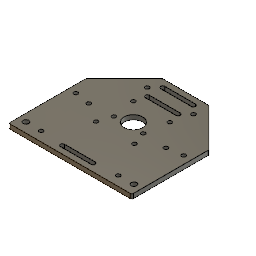
Motor_Mounting_Plate (Autodesk Fusion 360 design; units mm, degrees)
Autodesk Fusion 360 part; units mm, degrees
sketch "Sketch16" plane through (0, 0, 0) normal (0, 1, 0) x (1, 0, 0)
sketch "Sketch1" plane through (0, 0, 0) normal (0, 1, 0) x (1, 0, 0)
  line L0 (0, 0) -> (160, 0)
  line L1 (160, 0) -> (160, -150)
  line L2 (160, -150) -> (0, -150)
  line L3 (0, -150) -> (0, 0)
  line L4 (0, 0) -> (50, 0)
  line L5 (160, 0) -> (110, 0)
  line L6 (0, 0) -> (0, -50)
  line L7 (160, 0) -> (160, -50)
  line L8 (0, -50) -> (50, 0)
  line L9 (110, 0) -> (160, -50)
  dimension "d1" = 160
  dimension "d2" = 150
  dimension "d3" = 50
  dimension "d4" = 50
  dimension "d5" = 50
  measures "d1" distance of L0.start L0.end
  measures "d2" distance of L0.start L2.end
  measures "d3" distance of L0.end L5.end
  measures "d4" distance of L0.start L6.end
  measures "d5" distance of L0.end L7.end
extrude "Extrude1" add sketch "Sketch1" along normal blind 10 contours L0 L1 L2 L3 L8 L9
sketch "Sketch2" plane through (0, 10, 0) normal (0, 1, 0) x (-1, 0, 0)
  line L0 (-110, 0) -> (-50, 0)
  line L1 (-50, 0) -> (0, 50)
  line L2 (0, 50) -> (0, 150)
  line L3 (0, 150) -> (-160, 150)
  line L4 (-160, 150) -> (-160, 50)
  line L5 (-160, 50) -> (-110, 0)
  line L6 (0, 50) -> (-160, 50)
  line L7 (-80, 0) -> (-80, 150)
  circle A0 centre (-10, 72.7) radius 2.625
  circle A1 centre (-150.0228, 72.7) radius 2.625
  dimension "d10" = 5.25
  dimension "d13" = 5.25
  measures "d10" diameter of A0
  measures "d13" diameter of A1
extrude "Extrude2" cut sketch "Sketch2" against normal blind 200 contours A0 | A1
sketch "Sketch3" plane through (0, 10, 0) normal (0, 1, 0) x (-1, 0, 0)
  circle A0 centre (-10, 72.7) radius 2.625
  circle A1 centre (-150.0228, 72.7) radius 2.625
  line L0 (-110, 0) -> (-50, 0)
  line L1 (-50, 0) -> (0, 50)
  line L2 (0, 50) -> (0, 150)
  line L3 (0, 150) -> (-160, 150)
  line L4 (-160, 150) -> (-160, 50)
  line L5 (-160, 50) -> (-110, 0)
  line L6 (-80, 150) -> (-80, 68)
  circle A2 centre (-80, 68) radius 12
  dimension "d16" = 82
  dimension "d17" = 24
  measures "d16" distance of L6.start L6.end
  measures "d17" diameter of A2
extrude "Extrude3" cut sketch "Sketch3" against normal blind 45 contours A2
sketch "Sketch4" plane through (0, 10, 0) normal (0, 1, 0) x (-1, 0, 0)
  circle A0 centre (-80, 68) radius 12
  circle A1 centre (-10, 72.7) radius 2.625
  circle A2 centre (-150.0228, 72.7) radius 2.625
  line L0 (-110, 0) -> (-50, 0)
  line L1 (-50, 0) -> (0, 50)
  line L2 (0, 50) -> (0, 150)
  line L3 (0, 150) -> (-160, 150)
  line L4 (-160, 150) -> (-160, 50)
  line L5 (-160, 50) -> (-110, 0)
  line L6 (0, 150) -> (-30, 150)
  line L7 (-30, 150) -> (-30, 20)
  line L8 (-30, 150) -> (-30, 75.8)
  circle A3 centre (-30, 75.8) radius 2.625
  dimension "d20" = 30
  dimension "d21" = 130
  dimension "d22" = 74.2
  dimension "d23" = 5.25
  measures "d20" distance of L2.end L6.end
  measures "d21" distance of L6.end L7.end
  measures "d22" distance of L6.end L8.end
  measures "d23" diameter of A3
extrude "Extrude4" cut sketch "Sketch4" against normal blind 20 contours L7 L8 A3 | L7 L8 A3
sketch "Sketch5" plane through (0, 10, 0) normal (0, 1, 0) x (-1, 0, 0)
  circle A0 centre (-30, 75.8) radius 2.625
  circle A1 centre (-80, 68) radius 12
  circle A2 centre (-10, 72.7) radius 2.625
  circle A3 centre (-150.0228, 72.7) radius 2.625
  line L0 (-110, 0) -> (-50, 0)
  line L1 (-50, 0) -> (0, 50)
  line L2 (0, 50) -> (0, 150)
  line L3 (0, 150) -> (-160, 150)
  line L4 (-160, 150) -> (-160, 50)
  line L5 (-160, 50) -> (-110, 0)
  line L6 (0, 150) -> (-10, 150)
  line L7 (-10, 150) -> (-10, 137.3)
  line L8 (-160, 150) -> (-150, 150)
  line L9 (-150, 150) -> (-150, 137.3)
  circle A4 centre (-150, 137.3) radius 3.5685
  circle A5 centre (-10, 137.3) radius 3.5685
  dimension "d26" = 12.7
  dimension "d27" = 10
  dimension "d28" = 12.7
  dimension "d29" = 7.137
  dimension "d30" = 7.137
  measures "d26" distance of L6.end L7.end
  measures "d27" distance of L3.end L8.end
  measures "d28" distance of L8.end L9.end
  measures "d29" diameter of A4
  measures "d30" diameter of A5
extrude "Extrude5" cut sketch "Sketch5" against normal blind 12 contours A4 | A5
sketch "Sketch6" plane through (0, 10, 0) normal (0, 1, 0) x (-1, 0, 0)
  circle A0 centre (-10, 137.3) radius 3.5685
  circle A1 centre (-150, 137.3) radius 3.5685
  circle A2 centre (-30, 75.8) radius 2.625
  circle A3 centre (-80, 68) radius 12
  circle A4 centre (-10, 72.7) radius 2.625
  circle A5 centre (-150.0228, 72.7) radius 2.625
  line L0 (-110, 0) -> (-50, 0)
  line L1 (-50, 0) -> (0, 50)
  line L2 (0, 50) -> (0, 150)
  line L3 (0, 150) -> (-160, 150)
  line L4 (-160, 150) -> (-160, 50)
  line L5 (-160, 50) -> (-110, 0)
  line L6 (0, 150) -> (-30, 150)
  line L7 (-160, 150) -> (-130, 150)
  line L8 (-130, 150) -> (-130, 137.53)
  line L9 (-30, 150) -> (-30, 137.53)
  circle A6 centre (-30, 137.53) radius 2.625
  circle A7 centre (-130, 137.53) radius 2.625
  dimension "d33" = 30
  dimension "d34" = 30
  dimension "d35" = 12.47
  dimension "d36" = 12.47
  dimension "d37" = 5.25
  dimension "d38" = 5.25
  measures "d33" distance of L2.end L6.end
  measures "d34" distance of L3.end L7.end
  measures "d35" distance of L7.end L8.end
  measures "d36" distance of L6.end L9.end
  measures "d37" diameter of A6
  measures "d38" diameter of A7
extrude "Extrude6" cut sketch "Sketch6" against normal blind 20 contours A6 | A7
sketch "Sketch7" plane through (0, 10, 0) normal (0, 1, 0) x (-1, 0, 0)
  circle A0 centre (-30, 137.53) radius 2.625
  circle A1 centre (-130, 137.53) radius 2.625
  circle A2 centre (-10, 137.3) radius 3.5685
  circle A3 centre (-150, 137.3) radius 3.5685
  circle A4 centre (-30, 75.8) radius 2.625
  circle A5 centre (-80, 68) radius 12
  circle A6 centre (-10, 72.7) radius 2.625
  circle A7 centre (-150.0228, 72.7) radius 2.625
  line L0 (-110, 0) -> (-50, 0)
  line L1 (-50, 0) -> (0, 50)
  line L2 (0, 50) -> (0, 150)
  line L3 (0, 150) -> (-160, 150)
  line L4 (-160, 150) -> (-160, 50)
  line L5 (-160, 50) -> (-110, 0)
  line L6 (-130, 137.53) -> (-130, 60)
  line L7 (-30, 75.8) -> (-130, 75.8)
  circle A8 centre (-130, 75.8) radius 2.625
  dimension "d41" = 5.25
  measures "d41" diameter of A8
extrude "Extrude7" cut sketch "Sketch7" against normal blind 20 contours L6 L7 A8 | L6 A8 | L6 L7 A8
sketch "Sketch8" plane through (0, 10, 0) normal (0, 1, 0) x (-1, 0, 0)
  circle A0 centre (-130, 75.8) radius 2.625
  circle A1 centre (-30, 137.53) radius 2.625
  circle A2 centre (-130, 137.53) radius 2.625
  circle A3 centre (-10, 137.3) radius 3.5685
  circle A4 centre (-150, 137.3) radius 3.5685
  circle A5 centre (-30, 75.8) radius 2.625
  circle A6 centre (-80, 68) radius 12
  circle A7 centre (-10, 72.7) radius 2.625
  circle A8 centre (-150.0228, 72.7) radius 2.625
  line L0 (-110, 0) -> (-50, 0)
  line L1 (-50, 0) -> (0, 50)
  line L2 (0, 50) -> (0, 150)
  line L3 (0, 150) -> (-160, 150)
  line L4 (-160, 150) -> (-160, 50)
  line L5 (-160, 50) -> (-110, 0)
  line L6 (-80, 68) -> (-80, 150)
  line L7 (0, 150) -> (-99, 150)
  line L8 (0, 150) -> (-61, 150)
  line L9 (-61, 150) -> (-61, 74.1)
  line L10 (-99, 150) -> (-99, 74.1)
  circle A9 centre (-61, 74.1) radius 2.625
  circle A10 centre (-99, 74.1) radius 2.625
  dimension "d44" = 99
  dimension "d45" = 61
  dimension "d46" = 75.9
  dimension "d47" = 75.9
  dimension "d48" = 5.25
  dimension "d49" = 5.25
  measures "d44" distance of L2.end L7.end
  measures "d45" distance of L2.end L8.end
  measures "d46" distance of L8.end L9.end
  measures "d47" distance of L7.end L10.end
  measures "d48" diameter of A9
  measures "d49" diameter of A10
extrude "Extrude8" cut sketch "Sketch8" against normal blind 35 contours A9 | A10
sketch "Sketch9" plane through (0, 10, 0) normal (0, 1, 0) x (-1, 0, 0)
  circle A0 centre (-61, 74.1) radius 2.625
  circle A1 centre (-99, 74.1) radius 2.625
  circle A2 centre (-130, 75.8) radius 2.625
  circle A3 centre (-30, 137.53) radius 2.625
  circle A4 centre (-130, 137.53) radius 2.625
  circle A5 centre (-10, 137.3) radius 3.5685
  circle A6 centre (-150, 137.3) radius 3.5685
  circle A7 centre (-30, 75.8) radius 2.625
  circle A8 centre (-80, 68) radius 12
  circle A9 centre (-10, 72.7) radius 2.625
  circle A10 centre (-150.0228, 72.7) radius 2.625
  line L0 (-110, 0) -> (-50, 0)
  line L1 (-50, 0) -> (0, 50)
  line L2 (0, 50) -> (0, 150)
  line L3 (0, 150) -> (-160, 150)
  line L4 (-160, 150) -> (-160, 50)
  line L5 (-160, 50) -> (-110, 0)
  line L6 (0, 55) -> (-56.43, 55)
  line L7 (0, 55) -> (-103.57, 55)
  line L8 (-56.43, 55) -> (-56.43, 155)
  line L9 (-103.57, 55) -> (-103.57, 164.8084)
  line L10 (-103.57, 150) -> (-103.57, 44.43)
  line L11 (-56.43, 150) -> (-56.43, 44.43)
  circle A11 centre (-56.43, 44.43) radius 2.625
  circle A12 centre (-103.57, 44.43) radius 2.625
  dimension "d52" = 56.43
  dimension "d53" = 103.57
  dimension "d54" = 100
  dimension "d55" = 105.57
  dimension "d56" = 105.57
  dimension "d57" = 5.25
  dimension "d58" = 5.25
  measures "d52" distance of L6.start L6.end
  measures "d53" distance of L6.start L7.end
  measures "d54" distance of L6.end L8.end
  measures "d55" distance of L10.start L10.end
  measures "d56" distance of L11.start L11.end
  measures "d57" diameter of A11
  measures "d58" diameter of A12
extrude "Extrude9" cut sketch "Sketch9" against normal blind 12 contours A11 | A12
sketch "Sketch10" plane through (0, 10, 0) normal (0, 1, 0) x (-1, 0, 0)
  circle A0 centre (-103.57, 44.43) radius 2.625
  circle A1 centre (-56.43, 44.43) radius 2.625
  circle A2 centre (-61, 74.1) radius 2.625
  circle A3 centre (-99, 74.1) radius 2.625
  circle A4 centre (-130, 75.8) radius 2.625
  circle A5 centre (-30, 137.53) radius 2.625
  circle A6 centre (-130, 137.53) radius 2.625
  circle A7 centre (-10, 137.3) radius 3.5685
  circle A8 centre (-150, 137.3) radius 3.5685
  circle A9 centre (-30, 75.8) radius 2.625
  circle A10 centre (-80, 68) radius 12
  circle A11 centre (-10, 72.7) radius 2.625
  circle A12 centre (-150.0228, 72.7) radius 2.625
  line L0 (-110, 0) -> (-50, 0)
  line L1 (-50, 0) -> (0, 50)
  line L2 (0, 50) -> (0, 150)
  line L3 (0, 150) -> (-160, 150)
  line L4 (-160, 150) -> (-160, 50)
  line L5 (-160, 50) -> (-110, 0)
  line L6 (0, 150) -> (-55, 150)
  line L7 (0, 150) -> (-105, 150)
  line L8 (-55, 150) -> (-55, 91.57)
  line L9 (-105, 150) -> (-105, 91.57)
  circle A13 centre (-55, 91.57) radius 2.625
  circle A14 centre (-105, 91.57) radius 2.625
  dimension "d61" = 55
  dimension "d62" = 105
  dimension "d63" = 58.43
  dimension "d64" = 58.43
  dimension "d65" = 5.25
  dimension "d66" = 5.25
  measures "d61" distance of L2.end L6.end
  measures "d62" distance of L2.end L7.end
  measures "d63" distance of L6.end L8.end
  measures "d64" distance of L7.end L9.end
  measures "d65" diameter of A13
  measures "d66" diameter of A14
extrude "Extrude10" cut sketch "Sketch10" against normal blind 12 contours A13 | A14
sketch "Sketch11" plane through (0, 0, 0) normal (0, 1, 0) x (1, 0, 0)
sketch "Sketch12" plane through (0, 10, 0) normal (0, 1, 0) x (-1, 0, 0)
  circle A0 centre (-105, 91.57) radius 2.625
  circle A1 centre (-55, 91.57) radius 2.625
  circle A2 centre (-103.57, 44.43) radius 2.625
  circle A3 centre (-56.43, 44.43) radius 2.625
  circle A4 centre (-61, 74.1) radius 2.625
  circle A5 centre (-99, 74.1) radius 2.625
  circle A6 centre (-130, 75.8) radius 2.625
  circle A7 centre (-30, 137.53) radius 2.625
  circle A8 centre (-130, 137.53) radius 2.625
  circle A9 centre (-10, 137.3) radius 3.5685
  circle A10 centre (-150, 137.3) radius 3.5685
  circle A11 centre (-30, 75.8) radius 2.625
  circle A12 centre (-80, 68) radius 12
  circle A13 centre (-10, 72.7) radius 2.625
  circle A14 centre (-150.0228, 72.7) radius 2.625
  line L0 (-110, 0) -> (-50, 0)
  line L1 (-50, 0) -> (0, 50)
  line L2 (0, 50) -> (0, 150)
  line L3 (0, 150) -> (-160, 150)
  line L4 (-160, 150) -> (-160, 50)
  line L5 (-160, 50) -> (-110, 0)
  line L6 (0, 150) -> (-50, 150)
  line L7 (-50, 150) -> (-50, 20)
  line L8 (0, 150) -> (-110, 150)
  line L9 (-110, 150) -> (-110, 20)
  circle A15 centre (-50, 20) radius 2.625
  circle A16 centre (-110, 20) radius 2.625
  dimension "d69" = 50
  dimension "d70" = 130
  dimension "d71" = 110
  dimension "d72" = 130
  dimension "d73" = 5.25
  dimension "d74" = 5.25
  measures "d69" distance of L2.end L6.end
  measures "d70" distance of L6.end L7.end
  measures "d71" distance of L2.end L8.end
  measures "d72" distance of L8.end L9.end
  measures "d73" diameter of A15
  measures "d74" diameter of A16
extrude "Extrude11" cut sketch "Sketch12" against normal blind 20 contours A15 | A16
sketch "Sketch13" plane through (0, 10, 0) normal (0, 1, 0) x (-1, 0, 0)
  circle A0 centre (-110, 20) radius 2.625
  circle A1 centre (-50, 20) radius 2.625
  circle A2 centre (-105, 91.57) radius 2.625
  circle A3 centre (-55, 91.57) radius 2.625
  circle A4 centre (-103.57, 44.43) radius 2.625
  circle A5 centre (-56.43, 44.43) radius 2.625
  circle A6 centre (-61, 74.1) radius 2.625
  circle A7 centre (-99, 74.1) radius 2.625
  circle A8 centre (-130, 75.8) radius 2.625
  circle A9 centre (-30, 137.53) radius 2.625
  circle A10 centre (-130, 137.53) radius 2.625
  circle A11 centre (-10, 137.3) radius 3.5685
  circle A12 centre (-150, 137.3) radius 3.5685
  circle A13 centre (-30, 75.8) radius 2.625
  circle A14 centre (-80, 68) radius 12
  circle A15 centre (-10, 72.7) radius 2.625
  circle A16 centre (-150.0228, 72.7) radius 2.625
  line L0 (-110, 0) -> (-50, 0)
  line L1 (-50, 0) -> (0, 50)
  line L2 (0, 50) -> (0, 150)
  line L3 (0, 150) -> (-160, 150)
  line L4 (-160, 150) -> (-160, 50)
  line L5 (-160, 50) -> (-110, 0)
  line L6 (-80, 150) -> (-80, 10)
  line L7 (-100, 12.625) -> (-60, 12.625)
  line L8 (-60, 12.625) -> (-60, 7.375)
  line L9 (-60, 7.375) -> (-100, 7.375)
  line L10 (-100, 7.375) -> (-100, 12.625)
  line L11 (-100, 12.625) -> (-60, 7.375) construction
  line L12 (-60, 12.625) -> (-100, 7.375) construction
  line L13 (-80, 150) -> (-80, 30)
  line L14 (-60, 27.375) -> (-100, 27.375)
  line L15 (-100, 27.375) -> (-100, 32.625)
  line L16 (-100, 32.625) -> (-60, 32.625)
  line L17 (-60, 32.625) -> (-60, 27.375)
  line L18 (-60, 27.375) -> (-100, 32.625) construction
  line L19 (-100, 27.375) -> (-60, 32.625) construction
  line L20 (-80, 150) -> (-80, 140)
  line L21 (-100, 137.375) -> (-60, 137.375)
  line L22 (-60, 137.375) -> (-60, 142.625)
  line L23 (-60, 142.625) -> (-100, 142.625)
  line L24 (-100, 142.625) -> (-100, 137.375)
  line L25 (-100, 137.375) -> (-60, 142.625) construction
  line L26 (-60, 137.375) -> (-100, 142.625) construction
  point P0 (-80, 10)
  point P1 (-80, 30)
  point P2 (-80, 140)
  dimension "d77" = 140
  dimension "d78" = 40
  dimension "d79" = 5.25
  dimension "d80" = 120
  dimension "d81" = 40
  dimension "d82" = 5.25
  dimension "d83" = 10
  dimension "d84" = 40
  dimension "d85" = 5.25
  measures "d77" distance of L6.start P0
  measures "d78" distance of L8.end L9.end
  measures "d79" distance of L7.end L8.end
  measures "d80" distance of L6.start P1
  measures "d81" distance of L15.end L16.end
  measures "d82" distance of L14.end L15.end
  measures "d83" distance of L6.start P2
  measures "d84" distance of L22.end L23.end
  measures "d85" distance of L21.end L22.end
extrude "Extrude12" cut sketch "Sketch13" against normal blind 10 contours L6 L13 L20 L21 L22 L23 | L6 L13 L20 L21 L23 L24 | L6 L13 L14 L16 L17 | L6 L13 L14 L15 L16 | L7 L8 L9 L10
sketch "Sketch14" plane through (0, 10, 0) normal (0, 1, 0) x (-1, 0, 0)
  line L0 (-60, 12.625) -> (-60, 7.375)
  line L1 (-60, 7.375) -> (-100, 7.375)
  line L2 (-100, 7.375) -> (-100, 12.625)
  line L3 (-100, 12.625) -> (-60, 12.625)
  line L4 (-100, 27.375) -> (-100, 32.625)
  line L5 (-100, 32.625) -> (-60, 32.625)
  line L6 (-60, 32.625) -> (-60, 27.375)
  line L7 (-60, 27.375) -> (-100, 27.375)
  line L8 (-60, 137.375) -> (-100, 137.375)
  line L9 (-100, 137.375) -> (-100, 142.625)
  line L10 (-100, 142.625) -> (-60, 142.625)
  line L11 (-60, 142.625) -> (-60, 137.375)
  circle A0 centre (-110, 20) radius 2.625
  circle A1 centre (-50, 20) radius 2.625
  circle A2 centre (-105, 91.57) radius 2.625
  circle A3 centre (-55, 91.57) radius 2.625
  circle A4 centre (-103.57, 44.43) radius 2.625
  circle A5 centre (-56.43, 44.43) radius 2.625
  circle A6 centre (-61, 74.1) radius 2.625
  circle A7 centre (-99, 74.1) radius 2.625
  circle A8 centre (-130, 75.8) radius 2.625
  circle A9 centre (-30, 137.53) radius 2.625
  circle A10 centre (-130, 137.53) radius 2.625
  circle A11 centre (-10, 137.3) radius 3.5685
  circle A12 centre (-150, 137.3) radius 3.5685
  circle A13 centre (-30, 75.8) radius 2.625
  circle A14 centre (-80, 68) radius 12
  circle A15 centre (-10, 72.7) radius 2.625
  circle A16 centre (-150.0228, 72.7) radius 2.625
  line L12 (-110, 0) -> (-50, 0)
  line L13 (-50, 0) -> (0, 50)
  line L14 (0, 50) -> (0, 150)
  line L15 (0, 150) -> (-160, 150)
  line L16 (-160, 150) -> (-160, 50)
  line L17 (-160, 50) -> (-110, 0)
  circle A17 centre (-60, 140) radius 2.625
  circle A18 centre (-100, 140) radius 2.625
  dimension "d88" = 5.25
  dimension "d89" = 5.25
  measures "d88" diameter of A17
  measures "d89" diameter of A18
extrude "Extrude13" cut sketch "Sketch14" against normal blind 10 contours L11 A17 | L9 A18 picked at (-59.7535, 140.8396) picked at (-100.6233, 140.7327)
sketch "Sketch15" plane through (0, 10, 0) normal (0, 1, 0) x (-1, 0, 0)
  line L0 (-110, 0) -> (-50, 0)
  line L1 (-50, 0) -> (0, 50)
  line L2 (0, 50) -> (0, 150)
  line L3 (0, 150) -> (-160, 150)
  line L4 (-160, 150) -> (-160, 50)
  line L5 (-160, 50) -> (-110, 0)
  circle A0 centre (-150.0228, 72.7) radius 2.625
  circle A1 centre (-10, 72.7) radius 2.625
  circle A2 centre (-80, 68) radius 12
  circle A3 centre (-30, 75.8) radius 2.625
  circle A4 centre (-150, 137.3) radius 3.5685
  circle A5 centre (-10, 137.3) radius 3.5685
  circle A6 centre (-130, 137.53) radius 2.625
  circle A7 centre (-30, 137.53) radius 2.625
  circle A8 centre (-130, 75.8) radius 2.625
  circle A9 centre (-99, 74.1) radius 2.625
  circle A10 centre (-61, 74.1) radius 2.625
  circle A11 centre (-56.43, 44.43) radius 2.625
  circle A12 centre (-103.57, 44.43) radius 2.625
  circle A13 centre (-55, 91.57) radius 2.625
  circle A14 centre (-105, 91.57) radius 2.625
  circle A15 centre (-50, 20) radius 2.625
  circle A16 centre (-110, 20) radius 2.625
  line L6 (-100, 27.375) -> (-100, 32.625)
  line L7 (-100, 32.625) -> (-60, 32.625)
  line L8 (-60, 32.625) -> (-60, 27.375)
  line L9 (-60, 27.375) -> (-100, 27.375)
  line L10 (-60, 12.625) -> (-60, 7.375)
  line L11 (-60, 7.375) -> (-100, 7.375)
  line L12 (-100, 7.375) -> (-100, 12.625)
  line L13 (-100, 12.625) -> (-60, 12.625)
  arc A17 (-60, 137.375) -> (-60, 142.625) centre (-60, 140) ccw
  line L14 (-60, 137.375) -> (-100, 137.375)
  arc A18 (-100, 142.625) -> (-100, 137.375) centre (-100, 140) ccw
  line L15 (-100, 142.625) -> (-60, 142.625)
  circle A19 centre (-100, 30) radius 2.625
  circle A20 centre (-60, 30) radius 2.625
  circle A21 centre (-60, 10) radius 2.625
  circle A22 centre (-100, 10) radius 2.625
  dimension "d92" = 5.25
  dimension "d93" = 5.25
  dimension "d94" = 5.25
  dimension "d95" = 5.25
  measures "d92" diameter of A19
  measures "d93" diameter of A20
  measures "d94" diameter of A21
  measures "d95" diameter of A22
extrude "Extrude14" cut sketch "Sketch15" against normal blind 10 contours L6 A19 | L8 A20 | L10 A21 | L12 A22 picked at (-101.2414, 30.2238) picked at (-59.39, 30.8314) picked at (-59.7535, 10.8396) picked at (-101.2736, 9.5625)
fillet "Fillet1" radius 2 6 edges at (0, 5, 150) (160, 5, 150) (160, 5, 50) (110, 5, 0) (50, 5, 0) (0, 5, 50)
move_face "OffsetFaces3" offset -4 1 faces at (73.3333, 0, 107.9132)
sketch "Sketch18" plane through (0, 0, 150) normal (0, 0, 1) x (1, 0, 0)
  line L0 (158, 4) -> (158, 10)
  line L1 (158, 10) -> (2, 10)
  line L2 (2, 10) -> (2, 4)
  line L3 (2, 4) -> (158, 4)
